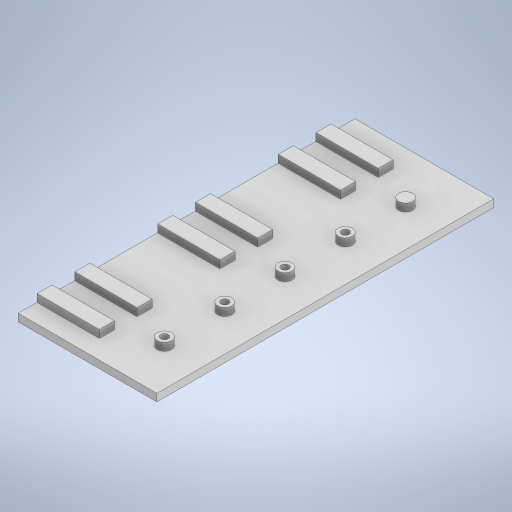
# Autodesk Inventor part: Podstawka
Saved by Autodesk Inventor 2024 (Build 280153000, 153)
## iProperties
Created: 2023-10-15
Part Number: Podstawka
Material: Generic
Document SubType Name: Modeling
Designer: Piter
Density: 1 g/cm^3
Appearance: Default
Author: Piter
Autodesk Inventor part; units mm, degrees
ref_plane "YZ Plane" through (0, 0, 0) normal (1, 0, 0) x (0, 1, 0)
ref_plane "XZ Plane" through (0, 0, 0) normal (0, 1, 0) x (-1, 0, 0)
ref_plane "XY Plane" through (0, 0, 0) normal (0, 0, 1) x (1, 0, 0)
sketch "Sketch1" plane through (0, 0, 0) normal (0, 1, 0) x (-1, 0, 0)
  line L0 (-12, 184.4696) -> (80, 184.4696)
  line L1 (80, 184.4696) -> (80, -38.9934)
  line L2 (80, -38.9934) -> (-12, -38.9934)
  line L3 (-12, -38.9934) -> (-12, 184.4696)
  point P0 (0, 0)
  dimension "d0" = 92
  dimension "d1" = 223.463
  constraints: 8 end point, 2 parallel, 1 horizontal, 1 perpendicular
  measures "d0" distance of L1.end L2.end
  measures "d1" distance of L0.end L1.end
extrude "Extrusion1" add sketch "Sketch1" along normal blind 5
sketch "Sketch2" plane through (0, 5, 0) normal (0, 1, 0) x (1, 0, 0)
  line L0 (-80, -184.4696) -> (12, -184.4696) projected
  line L1 (12, -184.4696) -> (-13, -184.4696)
  line L2 (-13, -184.4696) -> (-13, -154.4696)
  circle A0 centre (-13, -154.4696) radius 4.75
  line L3 (-13, -154.4696) -> (-13, -114.4696)
  line L4 (-13, -114.4696) -> (-13, -74.4696)
  line L5 (-13, -74.4696) -> (-13, -34.4696)
  circle A1 centre (-13, -114.4696) radius 4.75
  circle A2 centre (-13, -74.4696) radius 4.75
  circle A3 centre (-13, -34.4696) radius 4.75
  line L6 (-13, -34.4696) -> (-13, 5.5304)
  circle A4 centre (-13, 5.5304) radius 4.75
  point P0 (0, 0)
  dimension "d4" = 25
  dimension "d5" = 30
  dimension "d6" = 9.5
  dimension "d7" = 40
  dimension "d8" = 40
  dimension "d9" = 40
  dimension "d10" = 9.5
  dimension "d11" = 9.5
  dimension "d12" = 9.5
  dimension "d34" = 40
  dimension "d35" = 9.5
  constraints: 12 end point, 5 centre point, 5 coincident, 3 point on line, 2 vertical, 1 perpendicular
  measures "d4" distance of L0.end L1.end
  measures "d5" distance of L1.end L2.end
  measures "d6" diameter of A0
  measures "d7" distance of L3.start L3.end
  measures "d8" distance of L3.end L4.end
  measures "d9" distance of L4.end L5.end
  measures "d10" diameter of A1
  measures "d11" diameter of A2
  measures "d12" diameter of A3
  measures "d34" distance of L6.start L6.end
  measures "d35" diameter of A4
extrude "Extrusion2" add sketch "Sketch2" along normal blind 5
sketch "Sketch3" plane through (-13, 10, 154.4696) normal (0, 1, 0) x (1, 0, 0)
  circle A0 centre (0, 0) radius 2.5
  circle A1 centre (0, 0) radius 4.75 projected
  line L0 (0, 0) -> (0, 193.463)
  line L1 (25, 193.463) -> (-67, 193.463) projected
  circle A2 centre (0, 40) radius 2.5
  circle A3 centre (0, 80) radius 2.5
  circle A4 centre (0, 120) radius 2.5
  point P0 (13, 154.4696)
  dimension "d15" = 5
  dimension "d18" = 40
  constraints: 4 centre point, 2 end point, 2 vertical, 1 point on line, 6 other
  measures "d15" diameter of A0
  measures "d18" distance of A0.centre A2.centre
extrude "Extrusion3" cut sketch "Sketch3" against normal blind 3 contours A0 | A4 L0 | L0 A4 | A3 L0 | L0 A3 | A2 L0 | L0 A2
sketch "Sketch4" plane through (0, 5, 0) normal (0, 1, 0) x (1, 0, 0)
  circle A0 centre (-13, -154.4696) radius 2.5 projected
  line L0 (-13, -154.4696) -> (-80, -154.4696)
  line L1 (-80, 38.9934) -> (-80, -184.4696) projected
  line L2 (-40, -161.9696) -> (-80, -161.9696)
  line L3 (-80, -161.9696) -> (-80, -146.9696)
  line L4 (-80, -146.9696) -> (-40, -146.9696)
  line L5 (-40, -146.9696) -> (-40, -161.9696)
  line L6 (-40, -161.9696) -> (-80, -146.9696) construction
  line L7 (-80, -161.9696) -> (-40, -146.9696) construction
  line L8 (-80, -161.9696) -> (-38.6907, -161.9696)
  line L9 (-38.6907, -161.9696) -> (-38.6907, -171.9696)
  line L10 (-38.6907, -171.9696) -> (-80, -171.9696)
  line L11 (-80, -171.9696) -> (-80, -161.9696)
  line L12 (-80, -146.9696) -> (-38.6907, -146.9696)
  line L13 (-38.6907, -146.9696) -> (-38.6907, -136.9696)
  line L14 (-38.6907, -136.9696) -> (-80, -136.9696)
  line L15 (-80, -136.9696) -> (-80, -146.9696)
  point P0 (0, 0)
  point P1 (-60, -154.4696)
  point P2 (-40.5122, -103.5066)
  point P3 (-80, -136.9696)
  point P4 (-40.5122, -118.5066)
  point P5 (-80, -171.9696)
  point P6 (-40, -146.9696)
  point P7 (-40, -146.9696)
  point P8 (-40, -161.9696)
  dimension "d25" = 15
  dimension "d26" = 40
  dimension "d27" = 10
  dimension "d28" = 10
  constraints: 30 end point, 6 parallel, 4 horizontal, 4 point on line, 3 perpendicular, 2 midpoint
  measures "d25" distance of L2.end L3.end
  measures "d26" distance between parallel lines of L5 L1
  measures "d27" distance of L8.end L9.end
  measures "d28" distance of L13.end L12.end
extrude "Extrusion4" add sketch "Sketch4" along normal blind 5 contours L4 L1 L14 L13 L12 | L8 L9 L10 L1 L2
pattern_linear "Rectangular Pattern1" count 3 spacing 80 along (0, 0, -1) of "Extrusion4"
body "Solid1"
